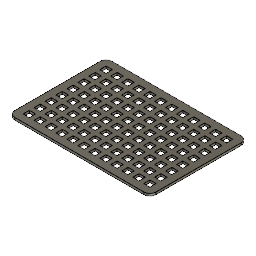
PCB_Gasket (Autodesk Fusion 360 design; units mm, degrees)
Autodesk Fusion 360 part; units mm, degrees
sketch "Sketch1" plane through (0, 0, 0) normal (0, 0, 1) x (1, 0, 0)
  line L0 (-53.0275, 40.0275) -> (53.0275, 40.0275)
  line L1 (58.0275, 35.0275) -> (58.0275, -35.0275)
  line L2 (53.0275, -40.0275) -> (-53.0275, -40.0275)
  line L3 (-58.0275, -35.0275) -> (-58.0275, 35.0275)
  line L4 (-58.0275, 40.0275) -> (58.0275, -40.0275) construction
  line L5 (58.0275, 40.0275) -> (-58.0275, -40.0275) construction
  line L6 (-58.38, -47.37) -> (-48.38, -47.37)
  arc A0 (-53.0275, 40.0275) -> (-58.0275, 35.0275) centre (-53.0275, 35.0275) ccw
  arc A1 (58.0275, 35.0275) -> (53.0275, 40.0275) centre (53.0275, 35.0275) ccw
  arc A2 (-58.0275, -35.0275) -> (-53.0275, -40.0275) centre (-53.0275, -35.0275) ccw
  arc A3 (53.0275, -40.0275) -> (58.0275, -35.0275) centre (53.0275, -35.0275) ccw
  line L7 (49.5, -31.5) -> (-49.5, -31.5)
  line L8 (-49.5, -31.5) -> (-49.5, 31.5)
  line L9 (-49.5, 31.5) -> (49.5, 31.5)
  line L10 (49.5, 31.5) -> (49.5, -31.5)
  line L11 (49.5, -31.5) -> (-49.5, 31.5) construction
  line L12 (-49.5, -31.5) -> (49.5, 31.5) construction
  line L13 (-46.9725, 28.9725) -> (-52.0275, 28.9725)
  line L14 (-52.0275, 28.9725) -> (-52.0275, 34.0275)
  line L15 (-52.0275, 34.0275) -> (-46.9725, 34.0275)
  line L16 (-46.9725, 34.0275) -> (-46.9725, 28.9725)
  line L17 (-46.9725, 28.9725) -> (-52.0275, 34.0275) construction
  line L18 (-52.0275, 28.9725) -> (-46.9725, 34.0275) construction
  line L19 (-43.0275, 28.9725) -> (-43.0275, 34.0275)
  line L20 (-37.9725, 28.9725) -> (-43.0275, 28.9725)
  line L21 (-37.9725, 34.0275) -> (-37.9725, 28.9725)
  line L22 (-43.0275, 34.0275) -> (-37.9725, 34.0275)
  line L23 (-34.0275, 28.9725) -> (-34.0275, 34.0275)
  line L24 (-28.9725, 28.9725) -> (-34.0275, 28.9725)
  line L25 (-28.9725, 34.0275) -> (-28.9725, 28.9725)
  line L26 (-34.0275, 34.0275) -> (-28.9725, 34.0275)
  line L27 (-25.0275, 28.9725) -> (-25.0275, 34.0275)
  line L28 (-19.9725, 28.9725) -> (-25.0275, 28.9725)
  line L29 (-19.9725, 34.0275) -> (-19.9725, 28.9725)
  line L30 (-25.0275, 34.0275) -> (-19.9725, 34.0275)
  line L31 (-16.0275, 28.9725) -> (-16.0275, 34.0275)
  line L32 (-10.9725, 28.9725) -> (-16.0275, 28.9725)
  line L33 (-10.9725, 34.0275) -> (-10.9725, 28.9725)
  line L34 (-16.0275, 34.0275) -> (-10.9725, 34.0275)
  line L35 (-7.0275, 28.9725) -> (-7.0275, 34.0275)
  line L36 (-1.9725, 28.9725) -> (-7.0275, 28.9725)
  line L37 (-1.9725, 34.0275) -> (-1.9725, 28.9725)
  line L38 (-7.0275, 34.0275) -> (-1.9725, 34.0275)
  line L39 (1.9725, 28.9725) -> (1.9725, 34.0275)
  line L40 (7.0275, 28.9725) -> (1.9725, 28.9725)
  line L41 (7.0275, 34.0275) -> (7.0275, 28.9725)
  line L42 (1.9725, 34.0275) -> (7.0275, 34.0275)
  line L43 (10.9725, 28.9725) -> (10.9725, 34.0275)
  line L44 (16.0275, 28.9725) -> (10.9725, 28.9725)
  line L45 (16.0275, 34.0275) -> (16.0275, 28.9725)
  line L46 (10.9725, 34.0275) -> (16.0275, 34.0275)
  line L47 (19.9725, 28.9725) -> (19.9725, 34.0275)
  line L48 (25.0275, 28.9725) -> (19.9725, 28.9725)
  line L49 (25.0275, 34.0275) -> (25.0275, 28.9725)
  line L50 (19.9725, 34.0275) -> (25.0275, 34.0275)
  line L51 (28.9725, 28.9725) -> (28.9725, 34.0275)
  line L52 (34.0275, 28.9725) -> (28.9725, 28.9725)
  line L53 (34.0275, 34.0275) -> (34.0275, 28.9725)
  line L54 (28.9725, 34.0275) -> (34.0275, 34.0275)
  line L55 (37.9725, 28.9725) -> (37.9725, 34.0275)
  line L56 (43.0275, 28.9725) -> (37.9725, 28.9725)
  line L57 (43.0275, 34.0275) -> (43.0275, 28.9725)
  line L58 (37.9725, 34.0275) -> (43.0275, 34.0275)
  line L59 (46.9725, 28.9725) -> (46.9725, 34.0275)
  line L60 (52.0275, 28.9725) -> (46.9725, 28.9725)
  line L61 (52.0275, 34.0275) -> (52.0275, 28.9725)
  line L62 (46.9725, 34.0275) -> (52.0275, 34.0275)
  line L63 (-52.0275, 19.9725) -> (-52.0275, 25.0275)
  line L64 (-46.9725, 19.9725) -> (-52.0275, 19.9725)
  line L65 (-46.9725, 25.0275) -> (-46.9725, 19.9725)
  line L66 (-52.0275, 25.0275) -> (-46.9725, 25.0275)
  line L67 (-43.0275, 19.9725) -> (-43.0275, 25.0275)
  line L68 (-37.9725, 19.9725) -> (-43.0275, 19.9725)
  line L69 (-37.9725, 25.0275) -> (-37.9725, 19.9725)
  line L70 (-43.0275, 25.0275) -> (-37.9725, 25.0275)
  line L71 (-34.0275, 19.9725) -> (-34.0275, 25.0275)
  line L72 (-28.9725, 19.9725) -> (-34.0275, 19.9725)
  line L73 (-28.9725, 25.0275) -> (-28.9725, 19.9725)
  line L74 (-34.0275, 25.0275) -> (-28.9725, 25.0275)
  line L75 (-25.0275, 19.9725) -> (-25.0275, 25.0275)
  line L76 (-19.9725, 19.9725) -> (-25.0275, 19.9725)
  line L77 (-19.9725, 25.0275) -> (-19.9725, 19.9725)
  line L78 (-25.0275, 25.0275) -> (-19.9725, 25.0275)
  line L79 (-16.0275, 19.9725) -> (-16.0275, 25.0275)
  line L80 (-10.9725, 19.9725) -> (-16.0275, 19.9725)
  line L81 (-10.9725, 25.0275) -> (-10.9725, 19.9725)
  line L82 (-16.0275, 25.0275) -> (-10.9725, 25.0275)
  line L83 (-7.0275, 19.9725) -> (-7.0275, 25.0275)
  line L84 (-1.9725, 19.9725) -> (-7.0275, 19.9725)
  line L85 (-1.9725, 25.0275) -> (-1.9725, 19.9725)
  line L86 (-7.0275, 25.0275) -> (-1.9725, 25.0275)
  line L87 (1.9725, 19.9725) -> (1.9725, 25.0275)
  line L88 (7.0275, 19.9725) -> (1.9725, 19.9725)
  line L89 (7.0275, 25.0275) -> (7.0275, 19.9725)
  line L90 (1.9725, 25.0275) -> (7.0275, 25.0275)
  line L91 (10.9725, 19.9725) -> (10.9725, 25.0275)
  line L92 (16.0275, 19.9725) -> (10.9725, 19.9725)
  line L93 (16.0275, 25.0275) -> (16.0275, 19.9725)
  line L94 (10.9725, 25.0275) -> (16.0275, 25.0275)
  line L95 (19.9725, 19.9725) -> (19.9725, 25.0275)
  line L96 (25.0275, 19.9725) -> (19.9725, 19.9725)
  line L97 (25.0275, 25.0275) -> (25.0275, 19.9725)
  line L98 (19.9725, 25.0275) -> (25.0275, 25.0275)
  line L99 (28.9725, 19.9725) -> (28.9725, 25.0275)
  line L100 (34.0275, 19.9725) -> (28.9725, 19.9725)
  line L101 (34.0275, 25.0275) -> (34.0275, 19.9725)
  line L102 (28.9725, 25.0275) -> (34.0275, 25.0275)
  line L103 (37.9725, 19.9725) -> (37.9725, 25.0275)
  line L104 (43.0275, 19.9725) -> (37.9725, 19.9725)
  line L105 (43.0275, 25.0275) -> (43.0275, 19.9725)
  line L106 (37.9725, 25.0275) -> (43.0275, 25.0275)
  line L107 (46.9725, 19.9725) -> (46.9725, 25.0275)
  line L108 (52.0275, 19.9725) -> (46.9725, 19.9725)
  line L109 (52.0275, 25.0275) -> (52.0275, 19.9725)
  line L110 (46.9725, 25.0275) -> (52.0275, 25.0275)
  line L111 (-52.0275, 10.9725) -> (-52.0275, 16.0275)
  line L112 (-46.9725, 10.9725) -> (-52.0275, 10.9725)
  line L113 (-46.9725, 16.0275) -> (-46.9725, 10.9725)
  line L114 (-52.0275, 16.0275) -> (-46.9725, 16.0275)
  line L115 (-43.0275, 10.9725) -> (-43.0275, 16.0275)
  line L116 (-37.9725, 10.9725) -> (-43.0275, 10.9725)
  line L117 (-37.9725, 16.0275) -> (-37.9725, 10.9725)
  line L118 (-43.0275, 16.0275) -> (-37.9725, 16.0275)
  line L119 (-34.0275, 10.9725) -> (-34.0275, 16.0275)
  line L120 (-28.9725, 10.9725) -> (-34.0275, 10.9725)
  line L121 (-28.9725, 16.0275) -> (-28.9725, 10.9725)
  line L122 (-34.0275, 16.0275) -> (-28.9725, 16.0275)
  line L123 (-25.0275, 10.9725) -> (-25.0275, 16.0275)
  line L124 (-19.9725, 10.9725) -> (-25.0275, 10.9725)
  line L125 (-19.9725, 16.0275) -> (-19.9725, 10.9725)
  line L126 (-25.0275, 16.0275) -> (-19.9725, 16.0275)
  line L127 (-16.0275, 10.9725) -> (-16.0275, 16.0275)
  line L128 (-10.9725, 10.9725) -> (-16.0275, 10.9725)
  line L129 (-10.9725, 16.0275) -> (-10.9725, 10.9725)
  line L130 (-16.0275, 16.0275) -> (-10.9725, 16.0275)
  line L131 (-7.0275, 10.9725) -> (-7.0275, 16.0275)
  line L132 (-1.9725, 10.9725) -> (-7.0275, 10.9725)
  line L133 (-1.9725, 16.0275) -> (-1.9725, 10.9725)
  line L134 (-7.0275, 16.0275) -> (-1.9725, 16.0275)
  line L135 (1.9725, 10.9725) -> (1.9725, 16.0275)
  line L136 (7.0275, 10.9725) -> (1.9725, 10.9725)
  line L137 (7.0275, 16.0275) -> (7.0275, 10.9725)
  line L138 (1.9725, 16.0275) -> (7.0275, 16.0275)
  line L139 (10.9725, 10.9725) -> (10.9725, 16.0275)
  line L140 (16.0275, 10.9725) -> (10.9725, 10.9725)
  line L141 (16.0275, 16.0275) -> (16.0275, 10.9725)
  line L142 (10.9725, 16.0275) -> (16.0275, 16.0275)
  line L143 (19.9725, 10.9725) -> (19.9725, 16.0275)
  line L144 (25.0275, 10.9725) -> (19.9725, 10.9725)
  line L145 (25.0275, 16.0275) -> (25.0275, 10.9725)
  line L146 (19.9725, 16.0275) -> (25.0275, 16.0275)
  line L147 (28.9725, 10.9725) -> (28.9725, 16.0275)
  line L148 (34.0275, 10.9725) -> (28.9725, 10.9725)
  line L149 (34.0275, 16.0275) -> (34.0275, 10.9725)
  line L150 (28.9725, 16.0275) -> (34.0275, 16.0275)
  line L151 (37.9725, 10.9725) -> (37.9725, 16.0275)
  line L152 (43.0275, 10.9725) -> (37.9725, 10.9725)
  line L153 (43.0275, 16.0275) -> (43.0275, 10.9725)
  line L154 (37.9725, 16.0275) -> (43.0275, 16.0275)
  line L155 (46.9725, 10.9725) -> (46.9725, 16.0275)
  line L156 (52.0275, 10.9725) -> (46.9725, 10.9725)
  line L157 (52.0275, 16.0275) -> (52.0275, 10.9725)
  line L158 (46.9725, 16.0275) -> (52.0275, 16.0275)
  line L159 (-52.0275, 1.9725) -> (-52.0275, 7.0275)
  line L160 (-46.9725, 1.9725) -> (-52.0275, 1.9725)
  line L161 (-46.9725, 7.0275) -> (-46.9725, 1.9725)
  line L162 (-52.0275, 7.0275) -> (-46.9725, 7.0275)
  line L163 (-43.0275, 1.9725) -> (-43.0275, 7.0275)
  line L164 (-37.9725, 1.9725) -> (-43.0275, 1.9725)
  line L165 (-37.9725, 7.0275) -> (-37.9725, 1.9725)
  line L166 (-43.0275, 7.0275) -> (-37.9725, 7.0275)
  line L167 (-34.0275, 1.9725) -> (-34.0275, 7.0275)
  line L168 (-28.9725, 1.9725) -> (-34.0275, 1.9725)
  line L169 (-28.9725, 7.0275) -> (-28.9725, 1.9725)
  line L170 (-34.0275, 7.0275) -> (-28.9725, 7.0275)
  line L171 (-25.0275, 1.9725) -> (-25.0275, 7.0275)
  line L172 (-19.9725, 1.9725) -> (-25.0275, 1.9725)
  line L173 (-19.9725, 7.0275) -> (-19.9725, 1.9725)
  line L174 (-25.0275, 7.0275) -> (-19.9725, 7.0275)
  line L175 (-16.0275, 1.9725) -> (-16.0275, 7.0275)
  line L176 (-10.9725, 1.9725) -> (-16.0275, 1.9725)
  line L177 (-10.9725, 7.0275) -> (-10.9725, 1.9725)
  line L178 (-16.0275, 7.0275) -> (-10.9725, 7.0275)
  line L179 (-7.0275, 1.9725) -> (-7.0275, 7.0275)
  line L180 (-1.9725, 1.9725) -> (-7.0275, 1.9725)
  line L181 (-1.9725, 7.0275) -> (-1.9725, 1.9725)
  line L182 (-7.0275, 7.0275) -> (-1.9725, 7.0275)
  line L183 (1.9725, 1.9725) -> (1.9725, 7.0275)
  line L184 (7.0275, 1.9725) -> (1.9725, 1.9725)
  line L185 (7.0275, 7.0275) -> (7.0275, 1.9725)
  line L186 (1.9725, 7.0275) -> (7.0275, 7.0275)
  line L187 (10.9725, 1.9725) -> (10.9725, 7.0275)
  line L188 (16.0275, 1.9725) -> (10.9725, 1.9725)
  line L189 (16.0275, 7.0275) -> (16.0275, 1.9725)
  line L190 (10.9725, 7.0275) -> (16.0275, 7.0275)
  line L191 (19.9725, 1.9725) -> (19.9725, 7.0275)
  line L192 (25.0275, 1.9725) -> (19.9725, 1.9725)
  line L193 (25.0275, 7.0275) -> (25.0275, 1.9725)
  line L194 (19.9725, 7.0275) -> (25.0275, 7.0275)
  line L195 (28.9725, 1.9725) -> (28.9725, 7.0275)
  line L196 (34.0275, 1.9725) -> (28.9725, 1.9725)
  line L197 (34.0275, 7.0275) -> (34.0275, 1.9725)
  line L198 (28.9725, 7.0275) -> (34.0275, 7.0275)
  line L199 (37.9725, 1.9725) -> (37.9725, 7.0275)
  line L200 (43.0275, 1.9725) -> (37.9725, 1.9725)
  line L201 (43.0275, 7.0275) -> (43.0275, 1.9725)
  line L202 (37.9725, 7.0275) -> (43.0275, 7.0275)
  line L203 (46.9725, 1.9725) -> (46.9725, 7.0275)
  line L204 (52.0275, 1.9725) -> (46.9725, 1.9725)
  line L205 (52.0275, 7.0275) -> (52.0275, 1.9725)
  line L206 (46.9725, 7.0275) -> (52.0275, 7.0275)
  line L207 (-52.0275, -7.0275) -> (-52.0275, -1.9725)
  line L208 (-46.9725, -7.0275) -> (-52.0275, -7.0275)
  line L209 (-46.9725, -1.9725) -> (-46.9725, -7.0275)
  line L210 (-52.0275, -1.9725) -> (-46.9725, -1.9725)
  line L211 (-43.0275, -7.0275) -> (-43.0275, -1.9725)
  line L212 (-37.9725, -7.0275) -> (-43.0275, -7.0275)
  line L213 (-37.9725, -1.9725) -> (-37.9725, -7.0275)
  line L214 (-43.0275, -1.9725) -> (-37.9725, -1.9725)
  line L215 (-34.0275, -7.0275) -> (-34.0275, -1.9725)
  line L216 (-28.9725, -7.0275) -> (-34.0275, -7.0275)
  line L217 (-28.9725, -1.9725) -> (-28.9725, -7.0275)
  line L218 (-34.0275, -1.9725) -> (-28.9725, -1.9725)
  line L219 (-25.0275, -7.0275) -> (-25.0275, -1.9725)
  line L220 (-19.9725, -7.0275) -> (-25.0275, -7.0275)
  line L221 (-19.9725, -1.9725) -> (-19.9725, -7.0275)
  line L222 (-25.0275, -1.9725) -> (-19.9725, -1.9725)
  line L223 (-16.0275, -7.0275) -> (-16.0275, -1.9725)
  line L224 (-10.9725, -7.0275) -> (-16.0275, -7.0275)
  line L225 (-10.9725, -1.9725) -> (-10.9725, -7.0275)
  line L226 (-16.0275, -1.9725) -> (-10.9725, -1.9725)
  line L227 (-7.0275, -7.0275) -> (-7.0275, -1.9725)
  line L228 (-1.9725, -7.0275) -> (-7.0275, -7.0275)
  line L229 (-1.9725, -1.9725) -> (-1.9725, -7.0275)
  line L230 (-7.0275, -1.9725) -> (-1.9725, -1.9725)
  line L231 (1.9725, -7.0275) -> (1.9725, -1.9725)
  line L232 (7.0275, -7.0275) -> (1.9725, -7.0275)
  line L233 (7.0275, -1.9725) -> (7.0275, -7.0275)
  line L234 (1.9725, -1.9725) -> (7.0275, -1.9725)
  line L235 (10.9725, -7.0275) -> (10.9725, -1.9725)
  line L236 (16.0275, -7.0275) -> (10.9725, -7.0275)
  line L237 (16.0275, -1.9725) -> (16.0275, -7.0275)
  line L238 (10.9725, -1.9725) -> (16.0275, -1.9725)
  line L239 (19.9725, -7.0275) -> (19.9725, -1.9725)
  line L240 (25.0275, -7.0275) -> (19.9725, -7.0275)
  line L241 (25.0275, -1.9725) -> (25.0275, -7.0275)
  line L242 (19.9725, -1.9725) -> (25.0275, -1.9725)
  line L243 (28.9725, -7.0275) -> (28.9725, -1.9725)
  line L244 (34.0275, -7.0275) -> (28.9725, -7.0275)
  line L245 (34.0275, -1.9725) -> (34.0275, -7.0275)
  line L246 (28.9725, -1.9725) -> (34.0275, -1.9725)
  line L247 (37.9725, -7.0275) -> (37.9725, -1.9725)
  line L248 (43.0275, -7.0275) -> (37.9725, -7.0275)
  line L249 (43.0275, -1.9725) -> (43.0275, -7.0275)
  line L250 (37.9725, -1.9725) -> (43.0275, -1.9725)
  line L251 (46.9725, -7.0275) -> (46.9725, -1.9725)
  line L252 (52.0275, -7.0275) -> (46.9725, -7.0275)
  line L253 (52.0275, -1.9725) -> (52.0275, -7.0275)
  line L254 (46.9725, -1.9725) -> (52.0275, -1.9725)
  line L255 (-52.0275, -16.0275) -> (-52.0275, -10.9725)
  line L256 (-46.9725, -16.0275) -> (-52.0275, -16.0275)
  line L257 (-46.9725, -10.9725) -> (-46.9725, -16.0275)
  line L258 (-52.0275, -10.9725) -> (-46.9725, -10.9725)
  line L259 (-43.0275, -16.0275) -> (-43.0275, -10.9725)
  line L260 (-37.9725, -16.0275) -> (-43.0275, -16.0275)
  line L261 (-37.9725, -10.9725) -> (-37.9725, -16.0275)
  line L262 (-43.0275, -10.9725) -> (-37.9725, -10.9725)
  line L263 (-34.0275, -16.0275) -> (-34.0275, -10.9725)
  line L264 (-28.9725, -16.0275) -> (-34.0275, -16.0275)
  line L265 (-28.9725, -10.9725) -> (-28.9725, -16.0275)
  line L266 (-34.0275, -10.9725) -> (-28.9725, -10.9725)
  line L267 (-25.0275, -16.0275) -> (-25.0275, -10.9725)
  line L268 (-19.9725, -16.0275) -> (-25.0275, -16.0275)
  line L269 (-19.9725, -10.9725) -> (-19.9725, -16.0275)
  line L270 (-25.0275, -10.9725) -> (-19.9725, -10.9725)
  line L271 (-16.0275, -16.0275) -> (-16.0275, -10.9725)
  line L272 (-10.9725, -16.0275) -> (-16.0275, -16.0275)
  line L273 (-10.9725, -10.9725) -> (-10.9725, -16.0275)
  line L274 (-16.0275, -10.9725) -> (-10.9725, -10.9725)
  line L275 (-7.0275, -16.0275) -> (-7.0275, -10.9725)
  line L276 (-1.9725, -16.0275) -> (-7.0275, -16.0275)
  line L277 (-1.9725, -10.9725) -> (-1.9725, -16.0275)
  line L278 (-7.0275, -10.9725) -> (-1.9725, -10.9725)
  line L279 (1.9725, -16.0275) -> (1.9725, -10.9725)
  line L280 (7.0275, -16.0275) -> (1.9725, -16.0275)
  line L281 (7.0275, -10.9725) -> (7.0275, -16.0275)
  line L282 (1.9725, -10.9725) -> (7.0275, -10.9725)
  line L283 (10.9725, -16.0275) -> (10.9725, -10.9725)
  line L284 (16.0275, -16.0275) -> (10.9725, -16.0275)
  line L285 (16.0275, -10.9725) -> (16.0275, -16.0275)
  line L286 (10.9725, -10.9725) -> (16.0275, -10.9725)
  line L287 (19.9725, -16.0275) -> (19.9725, -10.9725)
  line L288 (25.0275, -16.0275) -> (19.9725, -16.0275)
  line L289 (25.0275, -10.9725) -> (25.0275, -16.0275)
  line L290 (19.9725, -10.9725) -> (25.0275, -10.9725)
  line L291 (28.9725, -16.0275) -> (28.9725, -10.9725)
  line L292 (34.0275, -16.0275) -> (28.9725, -16.0275)
  line L293 (34.0275, -10.9725) -> (34.0275, -16.0275)
  line L294 (28.9725, -10.9725) -> (34.0275, -10.9725)
  line L295 (37.9725, -16.0275) -> (37.9725, -10.9725)
  line L296 (43.0275, -16.0275) -> (37.9725, -16.0275)
  line L297 (43.0275, -10.9725) -> (43.0275, -16.0275)
  line L298 (37.9725, -10.9725) -> (43.0275, -10.9725)
  line L299 (46.9725, -16.0275) -> (46.9725, -10.9725)
  line L300 (52.0275, -16.0275) -> (46.9725, -16.0275)
  line L301 (52.0275, -10.9725) -> (52.0275, -16.0275)
  line L302 (46.9725, -10.9725) -> (52.0275, -10.9725)
  line L303 (-52.0275, -25.0275) -> (-52.0275, -19.9725)
  line L304 (-46.9725, -25.0275) -> (-52.0275, -25.0275)
  line L305 (-46.9725, -19.9725) -> (-46.9725, -25.0275)
  line L306 (-52.0275, -19.9725) -> (-46.9725, -19.9725)
  line L307 (-43.0275, -25.0275) -> (-43.0275, -19.9725)
  line L308 (-37.9725, -25.0275) -> (-43.0275, -25.0275)
  line L309 (-37.9725, -19.9725) -> (-37.9725, -25.0275)
  line L310 (-43.0275, -19.9725) -> (-37.9725, -19.9725)
  line L311 (-34.0275, -25.0275) -> (-34.0275, -19.9725)
  line L312 (-28.9725, -25.0275) -> (-34.0275, -25.0275)
  line L313 (-28.9725, -19.9725) -> (-28.9725, -25.0275)
  line L314 (-34.0275, -19.9725) -> (-28.9725, -19.9725)
  line L315 (-25.0275, -25.0275) -> (-25.0275, -19.9725)
  line L316 (-19.9725, -25.0275) -> (-25.0275, -25.0275)
  line L317 (-19.9725, -19.9725) -> (-19.9725, -25.0275)
  line L318 (-25.0275, -19.9725) -> (-19.9725, -19.9725)
  line L319 (-16.0275, -25.0275) -> (-16.0275, -19.9725)
  line L320 (-10.9725, -25.0275) -> (-16.0275, -25.0275)
  line L321 (-10.9725, -19.9725) -> (-10.9725, -25.0275)
  line L322 (-16.0275, -19.9725) -> (-10.9725, -19.9725)
  line L323 (-7.0275, -25.0275) -> (-7.0275, -19.9725)
  line L324 (-1.9725, -25.0275) -> (-7.0275, -25.0275)
  line L325 (-1.9725, -19.9725) -> (-1.9725, -25.0275)
  line L326 (-7.0275, -19.9725) -> (-1.9725, -19.9725)
  line L327 (1.9725, -25.0275) -> (1.9725, -19.9725)
  line L328 (7.0275, -25.0275) -> (1.9725, -25.0275)
  line L329 (7.0275, -19.9725) -> (7.0275, -25.0275)
  line L330 (1.9725, -19.9725) -> (7.0275, -19.9725)
  line L331 (10.9725, -25.0275) -> (10.9725, -19.9725)
  line L332 (16.0275, -25.0275) -> (10.9725, -25.0275)
  line L333 (16.0275, -19.9725) -> (16.0275, -25.0275)
  line L334 (10.9725, -19.9725) -> (16.0275, -19.9725)
  line L335 (19.9725, -25.0275) -> (19.9725, -19.9725)
  line L336 (25.0275, -25.0275) -> (19.9725, -25.0275)
  line L337 (25.0275, -19.9725) -> (25.0275, -25.0275)
  line L338 (19.9725, -19.9725) -> (25.0275, -19.9725)
  line L339 (28.9725, -25.0275) -> (28.9725, -19.9725)
  line L340 (34.0275, -25.0275) -> (28.9725, -25.0275)
  line L341 (34.0275, -19.9725) -> (34.0275, -25.0275)
  line L342 (28.9725, -19.9725) -> (34.0275, -19.9725)
  line L343 (37.9725, -25.0275) -> (37.9725, -19.9725)
  line L344 (43.0275, -25.0275) -> (37.9725, -25.0275)
  line L345 (43.0275, -19.9725) -> (43.0275, -25.0275)
  line L346 (37.9725, -19.9725) -> (43.0275, -19.9725)
  line L347 (46.9725, -25.0275) -> (46.9725, -19.9725)
  line L348 (52.0275, -25.0275) -> (46.9725, -25.0275)
  line L349 (52.0275, -19.9725) -> (52.0275, -25.0275)
  line L350 (46.9725, -19.9725) -> (52.0275, -19.9725)
  line L351 (-52.0275, -34.0275) -> (-52.0275, -28.9725)
  line L352 (-46.9725, -34.0275) -> (-52.0275, -34.0275)
  line L353 (-46.9725, -28.9725) -> (-46.9725, -34.0275)
  line L354 (-52.0275, -28.9725) -> (-46.9725, -28.9725)
  line L355 (-43.0275, -34.0275) -> (-43.0275, -28.9725)
  line L356 (-37.9725, -34.0275) -> (-43.0275, -34.0275)
  line L357 (-37.9725, -28.9725) -> (-37.9725, -34.0275)
  line L358 (-43.0275, -28.9725) -> (-37.9725, -28.9725)
  line L359 (-34.0275, -34.0275) -> (-34.0275, -28.9725)
  line L360 (-28.9725, -34.0275) -> (-34.0275, -34.0275)
  line L361 (-28.9725, -28.9725) -> (-28.9725, -34.0275)
  line L362 (-34.0275, -28.9725) -> (-28.9725, -28.9725)
  line L363 (-25.0275, -34.0275) -> (-25.0275, -28.9725)
  line L364 (-19.9725, -34.0275) -> (-25.0275, -34.0275)
  line L365 (-19.9725, -28.9725) -> (-19.9725, -34.0275)
  line L366 (-25.0275, -28.9725) -> (-19.9725, -28.9725)
  line L367 (-16.0275, -34.0275) -> (-16.0275, -28.9725)
  line L368 (-10.9725, -34.0275) -> (-16.0275, -34.0275)
  line L369 (-10.9725, -28.9725) -> (-10.9725, -34.0275)
  line L370 (-16.0275, -28.9725) -> (-10.9725, -28.9725)
  line L371 (-7.0275, -34.0275) -> (-7.0275, -28.9725)
  line L372 (-1.9725, -34.0275) -> (-7.0275, -34.0275)
  line L373 (-1.9725, -28.9725) -> (-1.9725, -34.0275)
  line L374 (-7.0275, -28.9725) -> (-1.9725, -28.9725)
  line L375 (1.9725, -34.0275) -> (1.9725, -28.9725)
  line L376 (7.0275, -34.0275) -> (1.9725, -34.0275)
  line L377 (7.0275, -28.9725) -> (7.0275, -34.0275)
  line L378 (1.9725, -28.9725) -> (7.0275, -28.9725)
  line L379 (10.9725, -34.0275) -> (10.9725, -28.9725)
  line L380 (16.0275, -34.0275) -> (10.9725, -34.0275)
  line L381 (16.0275, -28.9725) -> (16.0275, -34.0275)
  line L382 (10.9725, -28.9725) -> (16.0275, -28.9725)
  line L383 (19.9725, -34.0275) -> (19.9725, -28.9725)
  line L384 (25.0275, -34.0275) -> (19.9725, -34.0275)
  line L385 (25.0275, -28.9725) -> (25.0275, -34.0275)
  line L386 (19.9725, -28.9725) -> (25.0275, -28.9725)
  line L387 (28.9725, -34.0275) -> (28.9725, -28.9725)
  line L388 (34.0275, -34.0275) -> (28.9725, -34.0275)
  line L389 (34.0275, -28.9725) -> (34.0275, -34.0275)
  line L390 (28.9725, -28.9725) -> (34.0275, -28.9725)
  line L391 (37.9725, -34.0275) -> (37.9725, -28.9725)
  line L392 (43.0275, -34.0275) -> (37.9725, -34.0275)
  line L393 (43.0275, -28.9725) -> (43.0275, -34.0275)
  line L394 (37.9725, -28.9725) -> (43.0275, -28.9725)
  line L395 (46.9725, -34.0275) -> (46.9725, -28.9725)
  line L396 (52.0275, -34.0275) -> (46.9725, -34.0275)
  line L397 (52.0275, -28.9725) -> (52.0275, -34.0275)
  line L398 (46.9725, -28.9725) -> (52.0275, -28.9725)
  point P0 (-57.3369, -42.2056)
  point P1 (-53.88, -84.89)
  point P2 (-49.5, 31.5)
  dimension "d1" = 116.055
  dimension "d2" = 80.055
  dimension "d15" = 5
  dimension "d16" = 5
  dimension "d17" = 5
  dimension "d18" = 5
  dimension "d19" = 99
  dimension "d20" = 63
  dimension "d21" = 5.055
  dimension "d22" = 5.055
  dimension "d25" = 99
  dimension "d26" = -63
  constraint perpendicular L0 L1
  constraint parallel L0 L2
  constraint parallel L1 L3
  constraint horizontal L0
  constraint horizontal L6
  constraint coincident L4.start L3
  constraint coincident L4.start L0
  constraint tangent L3 A0
  constraint tangent L0 A0
  constraint coincident L5.start L0
  constraint coincident L5.start L1
  constraint tangent L0 A1
  constraint tangent L1 A1
  constraint coincident L5.end L3
  constraint coincident L5.end L2
  constraint tangent L3 A2
  constraint tangent L2 A2
  constraint coincident L4.end L2
  constraint coincident L4.end L1
  constraint tangent L2 A3
  constraint tangent L1 A3
  constraint perpendicular L7 L8
  constraint parallel L7 L9
  constraint parallel L8 L10
  constraint horizontal L7
  constraint coincident L11 origin
  constraint coincident L12 origin
  constraint perpendicular L13 L14
  constraint parallel L13 L15
  constraint parallel L14 L16
  constraint horizontal L13
  constraint coincident L17 P2
  constraint coincident L18 P2
  constraint coincident P2 L8.end
  measures "d1" distance of L1 L3
  measures "d2" distance of L4.start L5.end
  measures "d15" radius of A0
  measures "d16" radius of A1
  measures "d17" radius of A2
  measures "d18" radius of A3
  measures "d19" distance of P2 L9.end
  measures "d20" distance of L7.end P2
  measures "d21" distance of L14.end L15.end
  measures "d22" distance of L13.end L14.end
extrude "Extrude1" add sketch "Sketch1" along normal blind 2 contours L0 L1 L2 L3 A0 A1 A2 A3 | L7 L8 L9 L10 L13 L16 L19 L20 L21 L23 L24 L25 L27 L28 L29 L31 L32 L33 L35 L36 L37 L39 L40 L41 L43 L44 L45 L47 L48 L49 L51 L52 L53 L55 L56 L57 L59 L60 L64 L65 L66 L107 L108 L110 L112 L113 L114 L155 L156 L158 L160 L161 L162 L203 L204 L206 L208 L209 L210 L251 L252 L254 L256 L257 L258 L299 L300 L302 L304 L305 L306 L347 L348 L350 L353 L354 L355 L357 L358 L359 L361 L362 L363 L365 L366 L367 L369 L370 L371 L373 L374 L375 L377 L378 L379 L381 L382 L383 L385 L386 L387 L389 L390 L391 L393 L394 L395 L398
